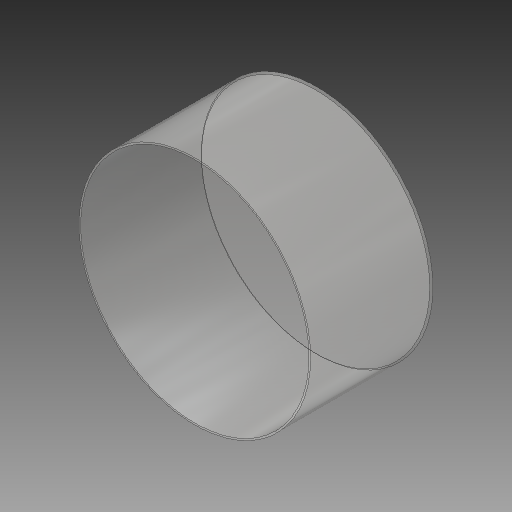
# Autodesk Inventor part: 使用タイヤ　プラ版部分
Saved by Autodesk Inventor 2017 (Build 210142000, 142)
## iProperties
Part Number: 使用タイヤ　プラ版部分
Material: PET プラスチック
Document SubType Name: Modeling
Designer: HISAAKI
Density: 1.541 g/cm^3
Appearance: ポリカーボネート - クリア
Author: HISAAKI
Autodesk Inventor part; units mm, degrees
ref_plane "YZ Plane" through (0, 0, 0) normal (1, 0, 0) x (0, 1, 0)
ref_plane "XZ Plane" through (0, 0, 0) normal (0, 1, 0) x (-1, 0, 0)
ref_plane "XY Plane" through (0, 0, 0) normal (0, 0, 1) x (1, 0, 0)
sketch "スケッチ1" plane through (0, 0, 0) normal (0, 0, 1) x (1, 0, 0)
  circle A0 centre (0, 0) radius 71
  dimension "d0" = 142
  constraints: 1 centre point, 1 coincident
  measures "d0" diameter of A0
extrude "押し出し1" add sketch "スケッチ1" along normal blind 75
shell "シェル1" thickness 1 removed faces 1 at (12.047, 0, 75)
